Autodesk Fusion 360 part; units mm, degrees
(part 4 of 6)
sketch "Sketch9" plane through (0, -25, 0) normal (0, 1, 0) x (-1, 0, 0)
  line L0 (-171.5, 52) -> (-171.5, 84)
  line L1 (-171.5, 84) -> (-111.5, 84)
  line L2 (-111.5, 84) -> (-111.5, 52)
  line L3 (-111.5, 52) -> (-171.5, 52)
  line L4 (-109, 89) -> (-139, 89)
  line L5 (-139, 89) -> (-139, 142)
  line L6 (-139, 142) -> (-109, 142)
  line L7 (-109, 142) -> (-109, 89)
  line L8 (-174, 89) -> (-174, 142)
  line L9 (-174, 142) -> (-144, 142)
  line L10 (-144, 142) -> (-144, 89)
  line L11 (-144, 89) -> (-174, 89)
  line L12 (-96, 65.5) -> (-93, 65.5)
  line L13 (-93, 65.5) -> (-93, 128.5)
  line L14 (-93, 128.5) -> (-60, 128.5)
  line L15 (-60, 128.5) -> (-60, 65.5)
  line L16 (-60, 65.5) -> (-57, 65.5)
  line L17 (-57, 65.5) -> (-57, 130.6162)
  line L18 (-57, 130.6162) -> (-54, 130.6162)
  line L19 (-54, 130.6162) -> (-54, 62.5)
  line L20 (-54, 62.5) -> (-99, 62.5)
  line L21 (-99, 62.5) -> (-99, 130.6162)
  line L22 (-99, 130.6162) -> (-96, 130.6162)
  line L23 (-96, 130.6162) -> (-96, 65.5)
  arc A0 (-52, 27) -> (-44, 35) centre (-52, 35) ccw
  line L24 (-44, 35) -> (-44, 159)
  arc A1 (-44, 159) -> (-52, 167) centre (-52, 159) ccw
  line L25 (-52, 167) -> (-176, 167)
  arc A2 (-176, 167) -> (-184, 159) centre (-176, 159) ccw
  line L26 (-184, 159) -> (-184, 35)
  arc A3 (-184, 35) -> (-176, 27) centre (-176, 35) ccw
  line L27 (-176, 27) -> (-52, 27)
  line L28 (-134, 27) -> (-94, 27)
  line L29 (-94, 27) -> (-94, 33)
  line L30 (-94, 33) -> (-134, 33)
  line L31 (-134, 33) -> (-134, 27)
  dimension "d68" = 6
  dimension "d70" = 50
  dimension "d71" = 50
  dimension "d103" = 40
  constraint horizontal L28
  constraint vertical L29
  constraint horizontal L30
  constraint vertical L31
  constraint coincident L27 L28.start
  measures "d68" distance of L28.start L30.end
  measures "d70" distance of L26 L31
  measures "d71" distance of L24 L29
  measures "d103" distance of L29.end L30.end
extrude "Extrude10" cut sketch "Sketch9" against normal blind 4 contours L27 L28 L29 L30 L31
sketch "Sketch10" plane through (0, -25, 0) normal (0, 1, 0) x (-1, 0, 0)
  line L0 (-134, 27) -> (-134, 33)
  line L1 (-134, 33) -> (-94, 33)
  line L2 (-94, 33) -> (-94, 27)
  line L3 (-94, 27) -> (-52, 27)
  arc A0 (-52, 27) -> (-44, 35) centre (-52, 35) ccw
  line L4 (-44, 35) -> (-44, 159)
  arc A1 (-44, 159) -> (-52, 167) centre (-52, 159) ccw
  line L5 (-52, 167) -> (-176, 167)
  arc A2 (-176, 167) -> (-184, 159) centre (-176, 159) ccw
  line L6 (-184, 159) -> (-184, 35)
  arc A3 (-184, 35) -> (-176, 27) centre (-176, 35) ccw
  line L7 (-176, 27) -> (-134, 27)
  line L8 (-96, 65.5) -> (-93, 65.5)
  line L9 (-93, 65.5) -> (-93, 128.5)
  line L10 (-93, 128.5) -> (-60, 128.5)
  line L11 (-60, 128.5) -> (-60, 65.5)
  line L12 (-60, 65.5) -> (-57, 65.5)
  line L13 (-57, 65.5) -> (-57, 130.6162)
  line L14 (-57, 130.6162) -> (-54, 130.6162)
  line L15 (-54, 130.6162) -> (-54, 62.5)
  line L16 (-54, 62.5) -> (-99, 62.5)
  line L17 (-99, 62.5) -> (-99, 130.6162)
  line L18 (-99, 130.6162) -> (-96, 130.6162)
  line L19 (-96, 130.6162) -> (-96, 65.5)
  line L20 (-174, 89) -> (-174, 142)
  line L21 (-174, 142) -> (-144, 142)
  line L22 (-144, 142) -> (-144, 89)
  line L23 (-144, 89) -> (-174, 89)
  line L24 (-109, 89) -> (-139, 89)
  line L25 (-139, 89) -> (-139, 142)
  line L26 (-139, 142) -> (-109, 142)
  line L27 (-109, 142) -> (-109, 89)
  line L28 (-171.5, 52) -> (-171.5, 84)
  line L29 (-171.5, 84) -> (-111.5, 84)
  line L30 (-111.5, 84) -> (-111.5, 52)
  line L31 (-111.5, 52) -> (-171.5, 52)
  line L32 (-184, 37) -> (-44, 37)
  line L33 (-44, 37) -> (-44, 33)
  line L34 (-44, 33) -> (-184, 33)
  line L35 (-184, 33) -> (-184, 37)
  dimension "d74" = 4
  constraint horizontal L32
  constraint vertical L33
  constraint horizontal L34
  constraint vertical L35
  constraint collinear L1 L34
  constraint collinear L4 L33
  constraint collinear L6 L35
  measures "d74" distance of L32 L34
extrude "Extrude11" add sketch "Sketch10" along normal blind 19 contours L1 A0 L4 L6 A3 L32 L33 L34 L35 | A3 L34 L35 | A0 L33 L34
sketch "Sketch11" plane through (0, -23, 0) normal (0, 1, 0) x (-1, 0, 0)
  line L0 (-174, 89) -> (-144, 89)
  line L1 (-144, 89) -> (-144, 142)
  line L2 (-144, 142) -> (-174, 142)
  line L3 (-174, 142) -> (-174, 89)
  line L4 (-169, 142) -> (-149, 142)
  line L5 (-149, 142) -> (-149, 132)
  line L6 (-149, 132) -> (-169, 132)
  line L7 (-169, 132) -> (-169, 142)
  line L8 (-134, 132) -> (-114, 132)
  line L9 (-114, 132) -> (-114, 142)
  line L10 (-114, 142) -> (-134, 142)
  line L11 (-134, 142) -> (-134, 132)
  line L12 (-171.5, 74) -> (-161.5, 74)
  line L13 (-161.5, 74) -> (-161.5, 62)
  line L14 (-161.5, 62) -> (-171.5, 62)
  line L15 (-171.5, 62) -> (-171.5, 74)
  line L16 (-171.5, 84) -> (-171.5, 52)
  line L17 (-111.5, 84) -> (-171.5, 84)
  line L18 (-171.5, 52) -> (-111.5, 52)
  line L19 (-111.5, 52) -> (-111.5, 84)
  line L20 (-111.5, 84) -> (-171.5, 84)
  line L21 (-171.5, 84) -> (-171.5, 52)
  line L22 (-109, 142) -> (-139, 142)
  line L23 (-109, 89) -> (-109, 142)
  line L24 (-139, 142) -> (-139, 89)
  dimension "d93" = 10
  dimension "d94" = 10
  dimension "d95" = 10
  dimension "d96" = 5
  dimension "d97" = 5
  dimension "d98" = 10
  dimension "d100" = 10
  dimension "d101" = 5
  dimension "d102" = 5
  constraint horizontal L4
  constraint vertical L5
  constraint horizontal L6
  constraint vertical L7
  constraint horizontal L8
  constraint vertical L9
  constraint horizontal L10
  constraint vertical L11
  constraint horizontal L12
  constraint vertical L13
  constraint horizontal L14
  constraint vertical L15
  constraint collinear L15 L16
  constraint collinear L4 L10
  constraint collinear L2 L4
  measures "d93" distance of L12.start L12.end
  measures "d94" distance of L12 L17
  measures "d95" distance of L14 L18
  measures "d96" distance of L1 L5
  measures "d97" distance of L3 L7
  measures "d98" distance of L4.end L5.end
  measures "d100" distance of L8 L22
  measures "d101" distance of L9 L23
  measures "d102" distance of L11 L24
extrude "Extrude12" cut sketch "Sketch11" against normal blind 6 contours L2 L4 L5 L6 L7 | L8 L9 L10 L11 L22 | L12 L13 L14 L15 L16 L21
sketch "Sketch12" plane through (0, -21, 0) normal (0, 1, 0) x (-1, 0, 0)
  line L0 (-57, 65.5) -> (-96, 65.5)
  line L1 (-96, 65.5) -> (-96, 130.6162)
  line L2 (-96, 130.6162) -> (-99, 130.6162)
  line L3 (-99, 130.6162) -> (-99, 62.5)
  line L4 (-99, 62.5) -> (-54, 62.5)
  line L5 (-54, 62.5) -> (-54, 130.6162)
  line L6 (-54, 130.6162) -> (-57, 130.6162)
  line L7 (-57, 130.6162) -> (-57, 65.5)
  line L8 (-99, 62.5) -> (-54, 62.5)
  line L9 (-54, 62.5) -> (-54, 75.5)
  line L10 (-54, 75.5) -> (-99, 75.5)
  line L11 (-99, 75.5) -> (-99, 62.5)
  dimension "d79" = 10
  constraint horizontal L8
  constraint vertical L9
  constraint horizontal L10
  constraint vertical L11
  constraint coincident L5 L9.end
  constraint coincident L3.end L4.start
  measures "d79" distance of L0 L10
extrude "Extrude13" add sketch "Sketch12" against normal blind 1 contours L0 L1 L3 L4 L5 L7 L8 L9 L10 L11 | L0 L1 L7 L10
sketch "Sketch13" plane through (0, -21, 0) normal (0, 1, 0) x (-1, 0, 0)
  line L0 (-54, 62.5) -> (-54, 130.6162)
  line L1 (-54, 130.6162) -> (-57, 130.6162)
  line L2 (-57, 130.6162) -> (-57, 75.5)
  line L3 (-57, 75.5) -> (-96, 75.5)
  line L4 (-96, 75.5) -> (-96, 130.6162)
  line L5 (-96, 130.6162) -> (-99, 130.6162)
  line L6 (-99, 130.6162) -> (-99, 62.5)
  line L7 (-99, 62.5) -> (-54, 62.5)
  line L8 (-99, 72) -> (-54, 72)
  line L9 (-54, 72) -> (-54, 70)
  line L10 (-54, 70) -> (-99, 70)
  line L11 (-99, 70) -> (-99, 72)
  dimension "d82" = 2
  constraint horizontal L8
  constraint vertical L9
  constraint horizontal L10
  constraint vertical L11
  constraint coincident L0 L9.end
  constraint coincident L6 L8.start
  measures "d82" distance of L8.end L9.end
extrude "Extrude14" add sketch "Sketch13" along normal blind 6 contours L0 L6 L8 L9 L10 L11
equation "d1 = 184 mm + ( ( 12 / 2 ) * 1 mm )"
equation "d2 = 140 mm + ( ( 2 * 27 ) * 1 mm )"
equation "d24 = 7.25 mm + ( ( 5.5 / 2 ) * 1 mm )"
equation "d25 = 7.25 mm + ( ( 5.5 / 2 ) * 1 mm )"
equation "d55 = ( ( 39 - 33 ) / 2 ) * 1 mm"
equation "d56 = ( ( 39 - 33 ) / 2 ) * 1 mm"
named bodies: "Electronics Holder"

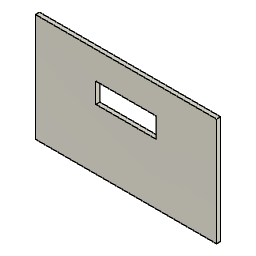
design "Unsorted Smarties Back Panel"
Autodesk Fusion 360 part; units mm, degrees
sketch "Unsorted Smarties Back" plane through (0, 0, 0) normal (0, 1, 0) x (1, 0, 0)
  line L0 (0, 0) -> (270, 0)
  line L1 (270, 0) -> (270, -161)
  line L2 (270, -161) -> (0, -161)
  line L3 (0, -161) -> (0, 0)
  dimension "d1" = 270
  dimension "d2" = 161
  constraint horizontal L0
  constraint vertical L1
  constraint horizontal L2
  constraint vertical L3
  constraint coincident L0.start L3.end
  measures "d1" distance of L0.start L0.end
  measures "d2" distance of L0.end L1.end
extrude "Extrude1" add sketch "Unsorted Smarties Back" along normal blind 6
sketch "Smartie Feed" plane through (0, 0, 0) normal (0, -1, 0) x (1, 0, 0)
  line L0 (270, 161) -> (0, 161)
  line L1 (0, 161) -> (0, 0)
  line L2 (0, 0) -> (270, 0)
  line L3 (270, 0) -> (270, 161)
  line L4 (90, 120) -> (180, 120)
  line L5 (180, 120) -> (180, 90)
  line L6 (180, 90) -> (90, 90)
  line L7 (90, 90) -> (90, 120)
  dimension "d6" = 90
  dimension "d7" = 90
  dimension "d8" = 41
  dimension "d9" = 30
  dimension "d12" = 90
  constraint horizontal L4
  constraint vertical L5
  constraint horizontal L6
  constraint vertical L7
  measures "d6" distance of L1 L7
  measures "d7" distance of L3 L5
  measures "d8" distance of L0 L4
  measures "d9" distance of L4.end L5.end
  measures "d12" distance of L5 L7
extrude "Extrude2" cut sketch "Smartie Feed" against normal blind 6 contours L4 L5 L6 L7
equation "mdfThickness = 6 mm"
equation "d4 = mdfThickness"
named bodies: "Unsorted Smarties Back Panel"

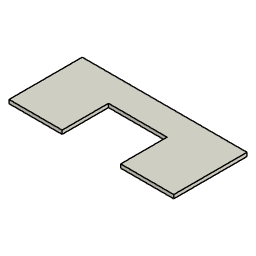
design "Colour Detection Mechanism Top Panel"
part number: 2025-05-13-09-48-31-121
Autodesk Fusion 360 part; units mm, degrees
sketch "Sorting Mechanism Top Panel" plane through (0, 0, 0) normal (0, 0, 1) x (1, 0, 0)
  line L0 (0, 0) -> (270, 0)
  line L1 (270, 0) -> (270, 120)
  line L2 (270, 120) -> (0, 120)
  line L3 (0, 120) -> (0, 0)
  dimension "d1" = 270
  dimension "d2" = 120
  constraint horizontal L0
  constraint vertical L1
  constraint horizontal L2
  constraint vertical L3
  constraint coincident L0.start L3.end
  measures "d1" distance of L0.start L0.end
  measures "d2" distance of L0.end L1.end
extrude "Extrude1" add sketch "Sorting Mechanism Top Panel" along normal blind 6
sketch "Smartie Hopper Hole" plane through (0, 0, 6) normal (0, 0, 1) x (-1, 0, 0)
  line L0 (0, -120) -> (0, 0)
  line L1 (0, 0) -> (-270, 0)
  line L2 (-270, 0) -> (-270, -120)
  line L3 (-270, -120) -> (0, -120)
  line L4 (-87, -76) -> (-183, -76)
  line L5 (-183, -76) -> (-183, 0)
  line L6 (-183, 0) -> (-87, 0)
  line L7 (-87, 0) -> (-87, -76)
  dimension "d7" = 96
  dimension "d9" = 76
  dimension "d10" = 87
  dimension "d11" = 87
  constraint horizontal L4
  constraint vertical L5
  constraint horizontal L6
  constraint vertical L7
  constraint collinear L1 L6
  measures "d7" distance of L4.start L4.end
  measures "d9" distance of L4.end L5.end
  measures "d10" distance of L0 L7
  measures "d11" distance of L2 L5
extrude "Extrude2" cut sketch "Smartie Hopper Hole" against normal blind 6 contours L1 L4 L5 L6 L7
equation "d3 = MDF_thickness"
equation "acrylic_thickness = 3 mm"
equation "MDF_thickness = 6 mm"
equation "d7 = smarties_hopper_width + 2 * acrylic_thickness"
equation "smarties_hopper_width = 90 mm"
equation "d9 = smarties_hopper_depth + 2 * acrylic_thickness"
equation "d10 = ( 270 mm - ( smarties_hopper_width + 2 * acrylic_thickness ) ) / 2"
equation "smarties_hopper_depth = 70 mm"
named bodies: "Sorting Mechanism Top Panel"

design "5 Volt Label"
Autodesk Fusion 360 part; units mm, degrees
sketch "Sticker" plane through (0, 0, 0) normal (0, 1, 0) x (1, 0, 0)
  line L0 (0, 0) -> (15, 0)
  line L1 (15, 0) -> (15, -12)
  line L2 (15, -12) -> (0, -12)
  line L3 (0, -12) -> (0, 0)
  dimension "d1" = 12
  dimension "d2" = 15
  constraint horizontal L0
  constraint vertical L1
  constraint horizontal L2
  constraint vertical L3
  constraint coincident L0.start L3.end
  measures "d1" distance of L0.end L1.end
  measures "d2" distance of L0.start L0.end
extrude "Extrude1" add sketch "Sticker" along normal blind 0.01 makes body 1
sketch "Text" plane through (0, 0, 0) normal (0, -1, 0) x (1, 0, 0)
  line L0 (15, 12) -> (0, 12)
  line L1 (0, 12) -> (0, 0)
  line L2 (0, 0) -> (15, 0)
  line L3 (15, 0) -> (15, 12)
  line L4 (0, 0) -> (15, 0) construction
  line L5 (15, 0) -> (15, 12) construction
  line L6 (15, 12) -> (0, 12) construction
  line L7 (0, 12) -> (0, 0) construction
  dimension "d5" = 5
  dimension "d8" = 0
  text T0 "5 V" font "Arial" height 5 align centre middle in box 15 x 12 at (0, 0) x (1, 0) y (0, 1) spacing 1 kerned
  constraint coincident L2.end
  constraint coincident L0.end
extrude "Extrude2" add sketch "Text" along normal blind 0.01 separate body text T0 makes body 2 at (4.016, 0, 8.2362) makes body 3 at (8.9069, 0, 7.2892)
equation "d8 = '5 V'"

design "Top Access Panel"
Autodesk Fusion 360 part; units mm, degrees
sketch "Top Access Panel" plane through (0, 0, 0) normal (0, 1, 0) x (1, 0, 0)
  line L0 (0, 0) -> (119, 0)
  line L1 (119, 0) -> (119, -89)
  line L2 (119, -89) -> (0, -89)
  line L3 (0, -89) -> (0, 0)
  dimension "d1" = 119
  dimension "d2" = 89
  constraint horizontal L0
  constraint vertical L1
  constraint horizontal L2
  constraint vertical L3
  constraint coincident L0.start L3.end
  measures "d1" distance of L0.start L0.end
  measures "d2" distance of L0.end L1.end
extrude "Extrude1" add sketch "Top Access Panel" along normal blind 6
fillet "Fillet1" radius 8 4 edges at (0, 3, 89) (119, 3, 89) (119, 3, 0) (0, 3, 0)
sketch "Handle" plane through (0, 6, 0) normal (0, 1, 0) x (-1, 0, 0)
  arc A0 (-8, 0) -> (0, 8) centre (-8, 8) ccw
  line L0 (0, 8) -> (0, 81)
  arc A1 (0, 81) -> (-8, 89) centre (-8, 81) ccw
  line L1 (-8, 89) -> (-111, 89)
  arc A2 (-111, 89) -> (-119, 81) centre (-111, 81) ccw
  line L2 (-119, 81) -> (-119, 8)
  arc A3 (-119, 8) -> (-111, 0) centre (-111, 8) ccw
  line L3 (-111, 0) -> (-8, 0)
  line L4 (-99, 0) -> (-20, 0)
  line L5 (-20, 0) -> (-20, 15)
  line L6 (-20, 15) -> (-99, 15)
  line L7 (-99, 15) -> (-99, 0)
  dimension "d16" = 15
  dimension "d17" = 20
  dimension "d18" = 20
  constraint horizontal L4
  constraint vertical L5
  constraint horizontal L6
  constraint vertical L7
  measures "d16" distance of L4 L6
  measures "d17" distance of L2 L7
  measures "d18" distance of L0 L5
extrude "Extrude3" cut sketch "Handle" against normal blind 6 contours L3 L4 L5 L6 L7
fillet "Fillet2" radius 15 2 edges at (99, 3, 15) (20, 3, 15)
sketch "Sketch4" plane through (0, 0, 0) normal (0, -1, 0) x (1, 0, 0)
  line L0 (35, 15) -> (84, 15)
  arc A0 (99, 0) -> (84, 15) centre (84, 0) ccw
  line L1 (99, 0) -> (111, 0)
  arc A1 (111, 0) -> (119, 8) centre (111, 8) ccw
  line L2 (119, 8) -> (119, 81)
  arc A2 (119, 81) -> (111, 89) centre (111, 81) ccw
  line L3 (111, 89) -> (8, 89)
  arc A3 (8, 89) -> (0, 81) centre (8, 81) ccw
  line L4 (0, 81) -> (0, 8)
  arc A4 (0, 8) -> (8, 0) centre (8, 8) ccw
  line L5 (8, 0) -> (20, 0)
  arc A5 (35, 15) -> (20, 0) centre (35, 0) ccw
  circle A6 centre (9.5, 79.237) radius 2.75
  circle A7 centre (109.5, 79.237) radius 2.75
  circle A8 centre (9.5, 9.237) radius 2.75
  circle A9 centre (109.5, 9.237) radius 2.75
  dimension "d23" = 5.5
  dimension "d24" = 5.5
  dimension "d25" = 5.5
  dimension "d26" = 5.5
  dimension "d27" = 9.5
  dimension "d28" = 9.5
  dimension "d29" = 9.5
  dimension "d30" = 9.5
  dimension "d31" = 9.763
  dimension "d32" = 9.763
  dimension "d33" = 9.237
  dimension "d34" = 9.237
  measures "d23" diameter of A6
  measures "d24" diameter of A7
  measures "d25" diameter of A8
  measures "d26" diameter of A9
  measures "d27" distance of L2 A9.centre
  measures "d28" distance of L4 A8.centre
  measures "d29" distance of L4 A6.centre
  measures "d30" distance of L2 A7.centre
  measures "d31" distance of L3 A6.centre
  measures "d32" distance of L3 A7.centre
  measures "d33" distance of L5 A8.centre
  measures "d34" distance of L1 A9.centre
extrude "Extrude4" cut sketch "Sketch4" against normal blind 1.5 contours A6 | A7 | A8 | A9
equation "mdfThickness = 6 mm"
equation "d4 = mdfThickness"
equation "filletRadius = 8 mm"
equation "d15 = filletRadius"
equation "d27 = 7.5 mm + ( ( 5.5 / 2 ) * 1 mm ) - 0.25 mm - 0.5 mm"
equation "d28 = 7.5 mm + ( ( 5.5 / 2 ) * 1 mm ) - 0.25 mm - 0.5 mm"
equation "d29 = 7.5 mm + ( ( 5.5 / 2 ) * 1 mm ) - 0.25 mm - 0.5 mm"
equation "d30 = 7.5 mm + ( ( 5.5 / 2 ) * 1 mm ) - 0.25 mm - 0.5 mm"
equation "d31 = 7.763 mm + ( ( 5.5 / 2 ) * 1 mm ) - 0.25 mm - 0.5 mm"
equation "d32 = 7.763 mm + ( ( 5.5 / 2 ) * 1 mm ) - 0.25 mm - 0.5 mm"
equation "d33 = 7.237 mm + ( ( 5.5 / 2 ) * 1 mm ) - 0.25 mm - 0.5 mm"
equation "d34 = 7.237 mm + ( ( 5.5 / 2 ) * 1 mm ) - 0.25 mm - 0.5 mm"

design "Name Sign Conduit"
Autodesk Fusion 360 part; units mm, degrees
sketch "16 mm x 16 mm conduit piping shape" plane through (0, 0, 0) normal (1, 0, 0) x (0, 1, 0)
  line L0 (0, 0) -> (16, 0)
  line L1 (16, 0) -> (16, 10)
  line L2 (16, 10) -> (14, 13.9)
  line L3 (14, 13.9) -> (13.1102, 13.4437)
  line L4 (13.1102, 13.4437) -> (15, 9.7585)
  line L5 (15, 9.7585) -> (15, 1)
  line L6 (15, 1) -> (1, 1)
  line L7 (1, 1) -> (1, 9.7585)
  line L8 (1, 9.7585) -> (2.8898, 13.4437)
  line L9 (2.8898, 13.4437) -> (2, 13.9)
  line L10 (2, 13.9) -> (0, 10)
  line L11 (0, 10) -> (0, 0)
  line L12 (0, 16) -> (16, 16)
  line L13 (0, 16) -> (0, 12)
  line L14 (0, 12) -> (1, 12)
  line L15 (1, 12) -> (1, 15)
  line L16 (1, 15) -> (15, 15)
  line L17 (15, 15) -> (15, 12)
  line L18 (15, 12) -> (16, 12)
  line L19 (16, 12) -> (16, 16)
  dimension "d1" = 1
  dimension "d2" = 16
  dimension "d3" = 1
  dimension "d4" = 1
  dimension "d7" = 10
  dimension "d8" = 10
  dimension "d9" = 16
  dimension "d10" = 1
  dimension "d11" = 1
  dimension "d12" = 1
  dimension "d13" = 4
  dimension "d14" = 4
  dimension "d15" = 16
  dimension "d16" = 2
  dimension "d17" = 2
  dimension "d18" = 1
  dimension "d19" = 1
  constraint coincident L0.start L11.end
  constraint horizontal L0
  constraint perpendicular L0 L1
  constraint perpendicular L2 L3
  constraint parallel L1 L5
  constraint perpendicular L5 L6
  constraint perpendicular L6 L7
  constraint perpendicular L0 L11
  constraint horizontal L12
  constraint perpendicular L12 L13
  constraint perpendicular L13 L14
  constraint perpendicular L14 L15
  constraint perpendicular L15 L16
  constraint perpendicular L16 L17
  constraint perpendicular L17 L18
  constraint perpendicular L12 L19
  constraint parallel L8 L10
  constraint parallel L2 L4
  constraint perpendicular L9 L10
  measures "d1" distance of L0 L6
  measures "d2" distance of L1 L11
  measures "d3" distance of L7 L11
  measures "d4" distance of L1 L5
  measures "d7" distance of L0.end L1.end
  measures "d8" distance of L10.end L0.start
  measures "d9" distance of L0 L12
  measures "d10" distance of L12 L16
  measures "d11" distance of L17 L19
  measures "d12" distance of L13 L15
  measures "d13" distance of L12.end L18.end
  measures "d14" distance of L12.start L13.end
  measures "d15" distance of L12.start L12.end
  measures "d16" distance of L1.end L2.end
  measures "d17" distance of L9.end L10.end
  measures "d18" distance of L2.end L3.end
  measures "d19" distance of L8.end L9.end
extrude "Extrude1" add sketch "16 mm x 16 mm conduit piping shape" along normal blind 161 makes body 1 at (107.3333, 5.3333, 16) makes body 2 at (53.6667, 5.3333, 0)
fillet "Fillet1" radius 0.3 18 edges at (80.5, 0, 16) (80.5, 16, 16) (80.5, 16, 12) (80.5, 0, 12) (80.5, 1, 12) (80.5, 15, 12) (80.5, 1, 15) (80.5, 15, 15) (80.5, 0, 10) (80.5, 16, 10) (80.5, 14, 13.9) (80.5, 13.1102, 13.4437) (80.5, 2, 13.9) (80.5, 2.8898, 13.4437) (80.5, 15, 1) (80.5, 1, 1) (80.5, 1, 9.7585) (80.5, 15, 9.7585) on bodies 1 2
equation "d1 = conduitThickness"
equation "d2 = conduitWidth"
equation "d3 = conduitThickness"
equation "d4 = conduitThickness"
equation "conduitThickness = 1 mm"
equation "conduitWidth = 16 mm"
equation "d9 = conduitWidth"
equation "d10 = conduitThickness"
equation "d11 = conduitThickness"
equation "d12 = conduitThickness"

design "Bottom Panel Opener"
Autodesk Fusion 360 part; units mm, degrees
sketch "Sketch1" plane through (0, 0, 0) normal (0, 0, 1) x (1, 0, 0)
  line L0 (-47.9346, 62.0575) -> (-70.9346, 62.0575)
  line L1 (-70.9346, 62.0575) -> (-70.9346, 122.0575)
  line L2 (-70.9346, 122.0575) -> (-47.9346, 122.0575)
  line L3 (-47.9346, 122.0575) -> (-47.9346, 62.0575)
  line L4 (-70.9346, 110) -> (-94.9346, 110)
  line L5 (-94.9346, 110) -> (-94.9346, 75)
  line L6 (-94.9346, 75) -> (-70.9346, 75)
  line L7 (-70.9346, 75) -> (-70.9346, 110)
  dimension "d1" = 35
  dimension "d3" = 60
  dimension "d4" = 24
  dimension "d10" = 23
  constraint horizontal L0
  constraint vertical L1
  constraint horizontal L2
  constraint vertical L3
  constraint horizontal L4
  constraint vertical L5
  constraint horizontal L6
  constraint vertical L7
  constraint coincident L1 L4.start
  measures "d1" distance of L4.end L5.end
  measures "d3" distance of L0.start L2.end
  measures "d4" distance of L4.start L4.end
  measures "d10" distance of L1 L3
extrude "Extrude1" add sketch "Sketch1" along normal blind 4
fillet "Fillet1" radius 4 2 edges at (-47.9346, 62.0575, 2) (-47.9346, 122.0575, 2)
fillet "Fillet1" radius 4 2 edges at (-94.9346, 75, 2) (-94.9346, 110, 2)

design "Front Panel"
Autodesk Fusion 360 part; units mm, degrees
sketch "Front Panel" plane through (0, 0, 0) normal (0, 1, 0) x (1, 0, 0)
  line L0 (0, 0) -> (270, 0)
  line L1 (270, 0) -> (270, -30)
  line L2 (258, -16) -> (12, -16)
  line L3 (0, -59) -> (0, 0)
  line L4 (12, -16) -> (12, -59)
  line L5 (12, -59) -> (0, -59)
  line L6 (258, -16) -> (258, -59)
  line L7 (258, -59) -> (270, -59)
  line L8 (270, -59) -> (270, -30)
  dimension "d1" = 270
  dimension "d3" = 43
  dimension "d4" = 12
  dimension "d5" = 12
  dimension "d10" = 16
  dimension "d11" = 43
  constraint horizontal L0
  constraint vertical L1
  constraint horizontal L2
  constraint vertical L3
  constraint coincident L0.start L3.end
  constraint vertical L4
  constraint horizontal L5
  constraint vertical L6
  constraint horizontal L7
  constraint vertical L8
  measures "d1" distance of L0.start L0.end
  measures "d3" distance of L2.end L4.end
  measures "d4" distance of L6.end L7.end
  measures "d5" distance of L4.end L3.start
  measures "d10" distance of L0 L2
  measures "d11" distance of L2 L7
extrude "Extrude1" add sketch "Front Panel" along normal blind 6
equation "mdfThickness = 6 mm"
equation "d7 = mdfThickness"
equation "d10 = 10 mm + mdfThickness"

design "Name Sign Bottom Connector"
Autodesk Fusion 360 part; units mm, degrees
sketch "Sketch1" plane through (0, 0, 0) normal (1, 0, 0) x (0, 1, 0)
  line L0 (25, 0) -> (0, 0)
  line L1 (0, 0) -> (-23.1302, 9.4864)
  line L2 (-23.1302, 9.4864) -> (-22.3713, 11.3368)
  line L3 (-22.3713, 11.3368) -> (0.3942, 2)
  line L4 (0.3942, 2) -> (25, 2)
  line L5 (25, 2) -> (25, 0)
  dimension "d1" = 157.7
  dimension "d2" = 2
  dimension "d3" = 2
  dimension "d4" = 25
  dimension "d5" = 25
  constraint coincident L0.end L1.start
  constraint horizontal L0
  constraint perpendicular L1 L2
  constraint perpendicular L2 L3
  constraint horizontal L4
  constraint perpendicular L0 L5
  measures "d1" angle of L3 L4
  measures "d2" distance of L0.start L4.end
  measures "d3" distance of L1.end L2.end
  measures "d4" distance of L0.end L1.end
  measures "d5" distance of L0.start L0.end
extrude "Extrude1" add sketch "Sketch1" against normal blind 15
sketch "Sketch2" plane through (0, 0, 2) normal (0, 0, 1) x (-1, 0, 0)
  line L0 (0, -0.3942) -> (0, -25)
  line L1 (0, -25) -> (15, -25)
  line L2 (15, -25) -> (15, -0.3942)
  line L3 (15, -0.3942) -> (0, -0.3942)
  circle A0 centre (5, -7.3942) radius 3
  circle A1 centre (10, -18) radius 3
  dimension "d8" = 6
  dimension "d9" = 6
  dimension "d10" = 5
  dimension "d11" = 5
  dimension "d12" = 7
  dimension "d14" = 7
  measures "d8" diameter of A0
  measures "d9" diameter of A1
  measures "d10" distance of L2 A1.centre
  measures "d11" distance of L0 A0.centre
  measures "d12" distance of L1 A1.centre
  measures "d14" distance of L3 A0.centre
sketch "Sketch3" plane through (0, 0.7589, 1.8504) normal (0, 0.379456, 0.92521) x (-1, 0, 0)
  line L0 (0, 25) -> (0, 0.3942)
  line L1 (0, 0.3942) -> (15, 0.3942)
  line L2 (15, 0.3942) -> (15, 25)
  line L3 (15, 25) -> (0, 25)
  circle A0 centre (10, 7.3942) radius 3
  circle A1 centre (5, 18) radius 3
  dimension "d15" = 6
  dimension "d16" = 6
  dimension "d17" = 5
  dimension "d18" = 5
  dimension "d19" = 7
  dimension "d20" = 7
  measures "d15" diameter of A0
  measures "d16" diameter of A1
  measures "d17" distance of L0 A1.centre
  measures "d18" distance of L2 A0.centre
  measures "d19" distance of L3 A1.centre
  measures "d20" distance of L1 A0.centre
extrude "Extrude2" cut sketch "Sketch3" against normal blind 2 contours A0 | A1
extrude "Extrude3" cut sketch "Sketch2" against normal blind 2 contours A0 | A1
fillet "Fillet1" radius 0.3 8 edges at (-2.203, -16.8986, 9.0923) (-7.203, -7.086, 5.0678) (-2.203, 6.3094, 2) (-7.203, 16.9152, 2) (-2.203, -15.6501, 6.4186) (-7.203, -5.8375, 2.3941) (-2.203, 8.479, 0) (-7.203, 19.0848, 0)

design "Smartie Arm"
Autodesk Fusion 360 part; units mm, degrees
sketch "Smartie Arm" plane through (0, 0, 0) normal (0, 0, 1) x (1, 0, 0)
  line L0 (0, 0) -> (95, 0)
  line L1 (95, 0) -> (95, 95)
  line L2 (95, 95) -> (0, 95)
  line L3 (0, 95) -> (0, 0)
  dimension "d6" = 95
  dimension "d15" = 95
  constraint horizontal L0
  constraint vertical L1
  constraint horizontal L2
  constraint vertical L3
  constraint coincident L0.start L3.end
  measures "d6" distance of L1.end L2.end
  measures "d15" distance of L0.end L1.end
extrude "Extrude1" add sketch "Smartie Arm" along normal blind 8
sketch "Smartie Hole" plane through (0, 0, 8) normal (0, 0, 1) x (-1, 0, 0)
  line L0 (0, -95) -> (0, 0)
  line L1 (0, 0) -> (-95, 0)
  line L2 (-95, 0) -> (-95, -95)
  line L3 (-95, -95) -> (0, -95)
  circle A0 centre (-15, -81) radius 9
  dimension "d5" = 18
  dimension "d8" = 15
  dimension "d9" = 80
  dimension "d14" = 14
  measures "d5" diameter of A0
  measures "d8" distance of L0 A0.centre
  measures "d9" distance of L2 A0.centre
  measures "d14" distance of L3 A0.centre
extrude "Extrude2" cut sketch "Smartie Hole" against normal blind 8 contours A0
fillet "Fillet1" radius 15 2 edges at (95, 95, 4) (0, 95, 4)
fillet "Fillet2" radius 15 2 edges at (0, 0, 4) (95, 0, 4)
sketch "Smartie Arm Arc" plane through (0, 0, 8) normal (0, 0, 1) x (-1, 0, 0)
  arc A0 (-80, 0) -> (-95, -15) centre (-80, -15) ccw
  line L0 (-95, -15) -> (-95, -80)
  arc A1 (-95, -80) -> (-80, -95) centre (-80, -80) ccw
  line L1 (-80, -95) -> (-15, -95)
  arc A2 (-15, -95) -> (0, -80) centre (-15, -80) ccw
  line L2 (0, -80) -> (0, -15)
  arc A3 (0, -15) -> (-15, 0) centre (-15, -15) ccw
  line L3 (-15, 0) -> (-80, 0)
  circle A4 centre (-15, -81) radius 9
  circle A5 centre (-15, -15) radius 80
  dimension "d16" = 15
  dimension "d17" = 15
  dimension "d18" = 160
  measures "d16" distance of L2.end A3.centre
  measures "d17" distance of L3 A3.centre
  measures "d18" diameter of A5
extrude "Extrude3" cut sketch "Smartie Arm Arc" against normal blind 8 contours L0 A1 L1 A5
equation "d14 = 16 mm - 2 mm"

design "Back Panel Support Bottom"
Autodesk Fusion 360 part; units mm, degrees
sketch "Back Panel Support Left " plane through (0, 0, 0) normal (1, 0, 0) x (0, 1, 0)
  line L0 (0, 0) -> (21, 0)
  line L1 (21, 0) -> (21, 21)
  line L2 (21, 21) -> (0, 21)
  line L3 (0, 21) -> (0, 0)
  dimension "d1" = 21
  dimension "d2" = 21
  constraint horizontal L0
  constraint vertical L1
  constraint horizontal L2
  constraint vertical L3
  constraint coincident L0.start L3.end
  measures "d1" distance of L0.end L1.end
  measures "d2" distance of L0.start L0.end
extrude "Extrude1" add sketch "Back Panel Support Left " along normal blind 228

design "Bottom Label"
Autodesk Fusion 360 part; units mm, degrees
sketch "Sticker" plane through (0, 0, 0) normal (0, 1, 0) x (1, 0, 0)
  line L0 (0, 0) -> (45, 0)
  line L1 (45, 0) -> (45, -12)
  line L2 (45, -12) -> (0, -12)
  line L3 (0, -12) -> (0, 0)
  dimension "d1" = 12
  dimension "d2" = 45
  constraint horizontal L0
  constraint vertical L1
  constraint horizontal L2
  constraint vertical L3
  constraint coincident L0.start L3.end
  measures "d1" distance of L0.end L1.end
  measures "d2" distance of L0.start L0.end
extrude "Extrude1" add sketch "Sticker" along normal blind 0.01 makes body 1
sketch "Text" plane through (0, 0, 0) normal (0, -1, 0) x (1, 0, 0)
  line L0 (45, 12) -> (0, 12)
  line L1 (0, 12) -> (0, 0)
  line L2 (0, 0) -> (45, 0)
  line L3 (45, 0) -> (45, 12)
  line L4 (0, 0) -> (45, 0) construction
  line L5 (45, 0) -> (45, 12) construction
  line L6 (45, 12) -> (0, 12) construction
  line L7 (0, 12) -> (0, 0) construction
  dimension "d5" = 5
  text T0 "Bottom" font "Arial" height 5 align centre middle in box 45 x 12 at (0, 0) x (1, 0) y (0, 1) spacing 1 kerned
  constraint coincident L2.end
  constraint coincident L0.end
extrude "Extrude2" add sketch "Text" along normal blind 0.01 separate body text T0 makes body 2 at (16.525, 0, 5.5613) makes body 3 at (28.3799, 0, 5.3338) makes body 4 at (24.291, 0, 5.5613) makes body 5 at (22.8695, 0, 5.244) makes body 6 at (20.9288, 0, 5.244) makes body 7 at (12.1373, 0, 5.9363)

design "6 Volt Label"
Autodesk Fusion 360 part; units mm, degrees
sketch "Sticker" plane through (0, 0, 0) normal (0, 1, 0) x (1, 0, 0)
  line L0 (0, 0) -> (15, 0)
  line L1 (15, 0) -> (15, -12)
  line L2 (15, -12) -> (0, -12)
  line L3 (0, -12) -> (0, 0)
  dimension "d1" = 12
  dimension "d2" = 15
  constraint horizontal L0
  constraint vertical L1
  constraint horizontal L2
  constraint vertical L3
  constraint coincident L0.start L3.end
  measures "d1" distance of L0.end L1.end
  measures "d2" distance of L0.start L0.end
extrude "Extrude1" add sketch "Sticker" along normal blind 0.01 makes body 1
sketch "Text" plane through (0, 0, 0) normal (0, -1, 0) x (1, 0, 0)
  line L0 (15, 12) -> (0, 12)
  line L1 (0, 12) -> (0, 0)
  line L2 (0, 0) -> (15, 0)
  line L3 (15, 0) -> (15, 12)
  line L4 (0, 0) -> (15, 0) construction
  line L5 (15, 0) -> (15, 12) construction
  line L6 (15, 12) -> (0, 12) construction
  line L7 (0, 12) -> (0, 0) construction
  dimension "d5" = 5
  dimension "d8" = 0
  text T0 "6 V" font "Arial" height 5 align centre middle in box 15 x 12 at (0, 0) x (1, 0) y (0, 1) spacing 1 kerned
  constraint coincident L2.end
  constraint coincident L0.end
extrude "Extrude2" add sketch "Text" along normal blind 0.01 separate body text T0 makes body 2 at (2.6313, 0, 6.1669) makes body 3 at (8.9205, 0, 7.2892)
equation "d8 = 6 V"

design "Female Header Pins"
Autodesk Fusion 360 part; units mm, degrees
sketch "Plastic casing" plane through (0, 0, 0) normal (0, 1, 0) x (1, 0, 0)
  line L0 (0, 0) -> (2.54, 0)
  line L1 (2.54, 0) -> (2.54, -8)
  line L2 (2.54, -8) -> (0, -8)
  line L3 (0, -8) -> (0, 0)
  dimension "d1" = 8
  dimension "d2" = 2.54
  constraint horizontal L0
  constraint vertical L1
  constraint horizontal L2
  constraint vertical L3
  constraint coincident L0.start L3.end
  measures "d1" distance of L0.end L1.end
  measures "d2" distance of L0.start L0.end
extrude "Extrude1" add sketch "Plastic casing" along normal blind 2.5 makes body 1
sketch "Hole" plane through (0, 0, 8) normal (0, 0, 1) x (-1, 0, 0)
  line L0 (0, 0) -> (-2.54, 0)
  line L1 (-2.54, 0) -> (-2.54, -2.5)
  line L2 (-2.54, -2.5) -> (0, -2.5)
  line L3 (0, -2.5) -> (0, 0)
  line L4 (-0.5, -2) -> (-2.04, -2)
  line L5 (-2.04, -2) -> (-2.04, -0.5)
  line L6 (-2.04, -0.5) -> (-0.5, -0.5)
  line L7 (-0.5, -0.5) -> (-0.5, -2)
  dimension "d6" = 0.5
  dimension "d7" = 0.5
  dimension "d8" = 0.5
  dimension "d9" = 0.5
  constraint horizontal L4
  constraint vertical L5
  constraint horizontal L6
  constraint vertical L7
  measures "d6" distance of L2 L4
  measures "d7" distance of L0 L6
  measures "d8" distance of L3 L7
  measures "d9" distance of L1 L5
extrude "Extrude2" cut sketch "Hole" against normal blind 7 contours L4 L5 L6 L7 bodies 1
sketch "Pin" plane through (0, 0, 0) normal (0, 0, 1) x (1, 0, 0)
  line L0 (2.54, 0) -> (0, 0)
  line L1 (0, 0) -> (0, 2.5)
  line L2 (0, 2.5) -> (2.54, 2.5)
  line L3 (2.54, 2.5) -> (2.54, 0)
  line L4 (0.945, 1.09) -> (1.595, 1.09)
  line L5 (1.595, 1.09) -> (1.595, 1.41)
  line L6 (1.595, 1.41) -> (0.945, 1.41)
  line L7 (0.945, 1.41) -> (0.945, 1.09)
  dimension "d12" = 0.65
  dimension "d13" = 0.32
  dimension "d14" = 0.945
  dimension "d15" = 0.945
  dimension "d16" = 1.09
  dimension "d17" = 1.09
  constraint horizontal L4
  constraint vertical L5
  constraint horizontal L6
  constraint vertical L7
  measures "d12" distance of L5.end L6.end
  measures "d13" distance of L4.end L5.end
  measures "d14" distance of L1 L7
  measures "d15" distance of L3 L5
  measures "d16" distance of L2 L6
  measures "d17" distance of L0 L4
extrude "Extrude3" add sketch "Pin" against normal blind 12 separate body contours L4 L5 L6 L7 makes body 2
chamfer "Chamfer1" distance 0.2 distance2 2 2 edges at (1.595, 1.25, -12) (0.945, 1.25, -12) measured on face at (1.1617, 1.3033, -12) measured on face at (1.1617, 1.3033, -12) on bodies 2
pattern_linear "R-Pattern1" count 15 spacing 2.54 along (1, 0, 0) of bodies 1 2 makes body 3 at (3.3867, 0, 2.6667) makes body 4 at (5.9267, 0, 2.6667) makes body 5 at (8.4667, 0, 2.6667) makes body 6 at (11.0067, 0, 2.6667) makes body 7 at (13.5467, 0, 2.6667) makes body 8 at (16.0867, 0, 2.6667) makes body 9 at (18.6267, 0, 2.6667) makes body 10 at (21.1667, 0, 2.6667) makes body 11 at (23.7067, 0, 2.6667) makes body 12 at (26.2467, 0, 2.6667) makes body 13 at (28.7867, 0, 2.6667) makes body 14 at (31.3267, 0, 2.6667) makes body 15 at (33.8667, 0, 2.6667) makes body 16 at (36.4067, 0, 2.6667) makes body 17 at (3.9183, 1.41, -3.3333) makes body 18 at (6.4583, 1.41, -3.3333) makes body 19 at (8.9983, 1.41, -3.3333) makes body 20 at (11.5383, 1.41, -3.3333) makes body 21 at (14.0783, 1.41, -3.3333) makes body 22 at (16.6183, 1.41, -3.3333) makes body 23 at (19.1583, 1.41, -3.3333) makes body 24 at (21.6983, 1.41, -3.3333) makes body 25 at (24.2383, 1.41, -3.3333) makes body 26 at (26.7783, 1.41, -3.3333) makes body 27 at (29.3183, 1.41, -3.3333) makes body 28 at (31.6417, 1.09, -3.3333) makes body 29 at (34.3983, 1.41, -3.3333) makes body 30 at (36.9383, 1.41, -3.3333)
equation "d14 = ( ( 2.54 - 0.65 ) / 2 ) * 1 mm"
equation "d16 = ( ( 2.5 - 0.32 ) / 2 ) * 1 mm"

design "12 Volt Label"
Autodesk Fusion 360 part; units mm, degrees
sketch "Sticker" plane through (0, 0, 0) normal (0, 1, 0) x (1, 0, 0)
  line L0 (0, 0) -> (15, 0)
  line L1 (15, 0) -> (15, -12)
  line L2 (15, -12) -> (0, -12)
  line L3 (0, -12) -> (0, 0)
  dimension "d1" = 12
  dimension "d2" = 15
  constraint horizontal L0
  constraint vertical L1
  constraint horizontal L2
  constraint vertical L3
  constraint coincident L0.start L3.end
  measures "d1" distance of L0.end L1.end
  measures "d2" distance of L0.start L0.end
extrude "Extrude1" add sketch "Sticker" along normal blind 0.01 makes body 1
sketch "Text" plane through (0, 0, 0) normal (0, -1, 0) x (1, 0, 0)
  line L0 (15, 12) -> (0, 12)
  line L1 (0, 12) -> (0, 0)
  line L2 (0, 0) -> (15, 0)
  line L3 (15, 0) -> (15, 12)
  line L4 (0, 0) -> (15, 0) construction
  line L5 (15, 0) -> (15, 12) construction
  line L6 (15, 12) -> (0, 12) construction
  line L7 (0, 12) -> (0, 0) construction
  dimension "d5" = 5
  dimension "d8" = 0
  text T0 "12 V" font "Arial" height 5 align centre middle in box 15 x 12 at (0, 0) x (1, 0) y (0, 1) spacing 1 kerned
  constraint coincident L2.end
  constraint coincident L0.end
extrude "Extrude2" add sketch "Text" along normal blind 0.01 separate body text T0 makes body 2 at (5.4445, 0, 3.6967) makes body 3 at (10.6139, 0, 7.2892) makes body 4 at (2.3602, 0, 6.4775)
equation "d8 = 12 V"

design "Savöx SH 0255 MG Micro Servo Horn"
Autodesk Fusion 360 part; units mm, degrees
sketch "Sketch1" plane through (0, 0, 0) normal (0, 0, 1) x (1, 0, 0)
  circle A0 centre (0, 0) radius 12
  dimension "d1" = 24
  constraint coincident A0.centre origin
  measures "d1" diameter of A0
extrude "Extrude1" add sketch "Sketch1" along normal blind 2
sketch "Sketch2" plane through (0, 0, 0) normal (0, 0, -1) x (1, 0, 0)
  circle A0 centre (0, 0) radius 12
  circle A1 centre (0, 0) radius 2.5
  circle A2 centre (0, 0) radius 3.5
  dimension "d4" = 5
  dimension "d5" = 7
  constraint concentric A0 A1
  constraint concentric A1 A2
  measures "d4" diameter of A1
  measures "d5" diameter of A2
extrude "Extrude2" add sketch "Sketch2" along normal blind 2 contours A2

design "Sorted Smarties Cover Connector Clip"
Autodesk Fusion 360 part; units mm, degrees
sketch "Sorted Smarties Cover Connector Clip" plane through (0, 0, 0) normal (0, 0, 1) x (1, 0, 0)
  line L0 (0, 0) -> (24, 0)
  line L1 (24, 0) -> (24, 17)
  line L2 (24, 17) -> (0, 17)
  line L3 (0, 17) -> (0, 0)
  dimension "d6" = 24
  dimension "d7" = 17
  constraint horizontal L0
  constraint vertical L1
  constraint horizontal L2
  constraint vertical L3
  constraint coincident L0.start L3.end
  measures "d6" distance of L0.start L0.end
  measures "d7" distance of L0.end L1.end
extrude "Extrude1" add sketch "Sorted Smarties Cover Connector Clip" along normal blind 4
sketch "Connecting Section" plane through (0, 0, 4) normal (0, 0, 1) x (-1, 0, 0)
  line L0 (0, -17) -> (0, 0)
  line L1 (0, 0) -> (-24, 0)
  line L2 (-24, 0) -> (-24, -17)
  line L3 (-24, -17) -> (0, -17)
  line L4 (0, -17) -> (-24, -17)
  line L5 (-24, -17) -> (-24, -12)
  line L6 (-24, -12) -> (0, -12)
  line L7 (0, -12) -> (0, -17)
  dimension "d5" = 5
  constraint horizontal L4
  constraint vertical L5
  constraint horizontal L6
  constraint vertical L7
  constraint coincident L2 L5.end
  constraint coincident L0.start L3.end
  measures "d5" distance of L2.end L5.end
extrude "Extrude2" add sketch "Connecting Section" along normal blind 9 contours L0 L2 L3 L4 L5 L6 L7
sketch "Sorted Smarties Cover Section" plane through (0, 0, 4) normal (0, 0, 1) x (-1, 0, 0)
  line L0 (-24, -12) -> (0, -12)
  line L1 (0, -12) -> (0, 0)
  line L2 (0, 0) -> (-24, 0)
  line L3 (-24, 0) -> (-24, -12)
  line L4 (0, 0) -> (-24, 0)
  line L5 (-24, 0) -> (-24, -4)
  line L6 (-24, -4) -> (0, -4)
  line L7 (0, -4) -> (0, 0)
  dimension "d8" = 4
  constraint horizontal L4
  constraint vertical L5
  constraint horizontal L6
  constraint vertical L7
  constraint coincident L3 L5.end
  constraint coincident L1.end L2.start
  measures "d8" distance of L4 L6
extrude "Extrude3" add sketch "Sorted Smarties Cover Section" along normal blind 15 contours L1 L2 L3 L4 L5 L6 L7
move_body "Move1" bodies 1 to x (-1, 0, 0) y (0, -1, 0) z (0, 0, 1) at (24, 17, 0)

design "Sorted Smarties Cover"
Autodesk Fusion 360 part; units mm, degrees
sketch "Sketch1" plane through (0, 0, 0) normal (0, 1, 0) x (1, 0, 0)
  line L0 (0, 0) -> (270, 0)
  line L1 (270, 0) -> (270, -264)
  line L2 (270, -264) -> (0, -264)
  line L3 (0, -264) -> (0, 0)
  dimension "d1" = 270
  dimension "d2" = 264
  constraint horizontal L0
  constraint vertical L1
  constraint horizontal L2
  constraint vertical L3
  constraint coincident L0.start L3.end
  measures "d1" distance of L1.end L2.end
  measures "d2" distance of L0.end L1.end
extrude "Extrude1" add sketch "Sketch1" along normal blind 6
sketch "Sketch2" plane through (0, 0, 0) normal (0, -1, 0) x (1, 0, 0)
  line L0 (270, 264) -> (0, 264)
  line L1 (0, 264) -> (0, 0)
  line L2 (0, 0) -> (270, 0)
  line L3 (270, 0) -> (270, 264)
  line L4 (25.625, 231.1665) -> (43.625, 231.1665)
  line L5 (43.625, 231.1665) -> (43.625, 213.1665)
  line L6 (43.625, 213.1665) -> (25.625, 213.1665)
  line L7 (25.625, 213.1665) -> (25.625, 231.1665)
  line L8 (91.875, 231.1665) -> (109.875, 231.1665)
  line L9 (109.875, 231.1665) -> (109.875, 213.1665)
  line L10 (109.875, 213.1665) -> (91.875, 213.1665)
  line L11 (91.875, 213.1665) -> (91.875, 231.1665)
  line L12 (160.125, 231.1665) -> (178.125, 231.1665)
  line L13 (178.125, 231.1665) -> (178.125, 213.1665)
  line L14 (178.125, 213.1665) -> (160.125, 213.1665)
  line L15 (160.125, 213.1665) -> (160.125, 231.1665)
  line L16 (226.375, 231.1665) -> (244.375, 231.1665)
  line L17 (244.375, 231.1665) -> (244.375, 213.1665)
  line L18 (244.375, 213.1665) -> (226.375, 213.1665)
  line L19 (226.375, 213.1665) -> (226.375, 231.1665)
  line L20 (25.625, 111.6665) -> (43.625, 111.6665)
  line L21 (43.625, 111.6665) -> (43.625, 93.6665)
  line L22 (43.625, 93.6665) -> (25.625, 93.6665)
  line L23 (25.625, 93.6665) -> (25.625, 111.6665)
  line L24 (91.875, 111.6665) -> (109.875, 111.6665)
  line L25 (109.875, 111.6665) -> (109.875, 93.6665)
  line L26 (109.875, 93.6665) -> (91.875, 93.6665)
  line L27 (91.875, 93.6665) -> (91.875, 111.6665)
  line L28 (160.125, 111.6665) -> (178.125, 111.6665)
  line L29 (178.125, 111.6665) -> (178.125, 93.6665)
  line L30 (178.125, 93.6665) -> (160.125, 93.6665)
  line L31 (160.125, 93.6665) -> (160.125, 111.6665)
  line L32 (226.375, 111.6665) -> (244.375, 111.6665)
  line L33 (244.375, 111.6665) -> (244.375, 93.6665)
  line L34 (244.375, 93.6665) -> (226.375, 93.6665)
  line L35 (226.375, 93.6665) -> (226.375, 111.6665)
  dimension "d5" = 18
  dimension "d6" = 18
  dimension "d7" = 18
  dimension "d8" = 18
  dimension "d9" = 18
  dimension "d10" = 18
  dimension "d11" = 270
  dimension "d12" = 264
  dimension "d13" = 25.625
  dimension "d17" = 32.8335
  dimension "d18" = 152.3335
  dimension "d19" = 48.25
  dimension "d22" = 48.25
  dimension "d24" = 25.625
  constraint horizontal L4
  constraint vertical L5
  constraint horizontal L6
  constraint vertical L7
  constraint horizontal L8
  constraint vertical L9
  constraint horizontal L10
  constraint vertical L11
  constraint horizontal L12
  constraint vertical L13
  constraint horizontal L14
  constraint vertical L15
  constraint horizontal L16
  constraint vertical L17
  constraint horizontal L18
  constraint vertical L19
  constraint collinear L12 L16
  constraint collinear L8 L12
  constraint collinear L4 L8
  constraint collinear L14 L18
  constraint collinear L10 L14
  constraint collinear L6 L10
  constraint horizontal L20
  constraint vertical L21
  constraint horizontal L22
  constraint vertical L23
  constraint horizontal L24
  constraint vertical L25
  constraint horizontal L26
  constraint vertical L27
  constraint horizontal L28
  constraint vertical L29
  constraint horizontal L30
  constraint vertical L31
  constraint horizontal L32
  constraint vertical L33
  constraint horizontal L34
  constraint vertical L35
  constraint collinear L7 L23
  constraint collinear L5 L21
  constraint collinear L11 L27
  constraint collinear L9 L25
  constraint collinear L15 L31
  constraint collinear L13 L29
  constraint collinear L19 L35
  constraint collinear L17 L33
  constraint collinear L20 L24
  constraint collinear L24 L28
  constraint collinear L28 L32
  constraint collinear L22 L26
  constraint collinear L26 L30
  constraint collinear L30 L34
  measures "d5" distance of L5.end L6.end
  measures "d6" distance of L9.end L10.end
  measures "d7" distance of L13.end L14.end
  measures "d8" distance of L17.end L18.end
  measures "d9" distance of L4.start L6.end
  measures "d10" distance of L20.start L22.end
  measures "d11" distance of L0.start L0.end
  measures "d12" distance of L0.start L2.end
  measures "d13" distance of L1 L7
  measures "d17" distance of L0 L4
  measures "d18" distance of L0 L20
  measures "d19" distance of L5 L11
  measures "d22" distance of L13 L19
  measures "d24" distance of L3 L17
extrude "Extrude2" cut sketch "Sketch2" against normal blind 6 contours L4 L5 L6 L7 | L8 L9 L10 L11 | L12 L13 L14 L15 | L16 L17 L18 L19 | L20 L21 L22 L23 | L24 L25 L26 L27 | L28 L29 L30 L31 | L32 L33 L34 L35
equation "d13 = 3 mm + ( ( 63.25 / 2 ) * 1 mm ) - ( ( 18 / 2 ) * 1 mm )"
equation "d17 = 3 mm + ( ( 77.667 / 2 ) * 1 mm ) - ( ( 18 / 2 ) * 1 mm )"
equation "d18 = 122.5 mm + ( ( 77.667 / 2 ) * 1 mm ) - ( ( 18 / 2 ) * 1 mm )"
equation "d19 = 3 mm + 63.25 mm - 18 mm"
equation "d22 = 3 mm + 63.25 mm - 18 mm"
equation "d24 = 3 mm + ( ( 63.25 / 2 ) * 1 mm ) - ( ( 18 / 2 ) * 1 mm )"

design "Smartie Feed"
Autodesk Fusion 360 part; units mm, degrees
sketch "Smartie Feed" plane through (0, 0, 0) normal (0, 0, 1) x (1, 0, 0)
  line L0 (0, 0) -> (209, 0)
  line L1 (209, 0) -> (209, 21)
  line L2 (209, 21) -> (0, 21)
  line L3 (0, 21) -> (0, 0)
  dimension "d1" = 209
  dimension "d2" = 21
  constraint horizontal L0
  constraint vertical L1
  constraint horizontal L2
  constraint vertical L3
  constraint coincident L0.start L3.end
  measures "d1" distance of L0.start L0.end
  measures "d2" distance of L0.end L1.end
extrude "Extrude1" add sketch "Smartie Feed" along normal blind 187
sketch "Outlet" plane through (0, 0, 0) normal (0, -1, 0) x (1, 0, 0)
  line L0 (0, 0) -> (209, 0)
  line L1 (209, 0) -> (209, 187)
  line L2 (209, 187) -> (0, 187)
  line L3 (0, 187) -> (0, 0)
  line L4 (69, 146) -> (159, 146)
  line L5 (159, 146) -> (159, 116)
  line L6 (159, 116) -> (69, 116)
  line L7 (69, 116) -> (69, 146)
  dimension "d31" = 30
  dimension "d32" = 90
  dimension "d33" = 69
  dimension "d34" = 50
  dimension "d35" = 41
  constraint horizontal L4
  constraint vertical L5
  constraint horizontal L6
  constraint vertical L7
  measures "d31" distance of L4.end L5.end
  measures "d32" distance of L4.start L4.end
  measures "d33" distance of L3 L7
  measures "d34" distance of L1 L5
  measures "d35" distance of L2 L4
sketch "Inlet" plane through (0, 21, 0) normal (0, 1, 0) x (-1, 0, 0)
  line L0 (-209, 0) -> (0, 0)
  line L1 (0, 0) -> (0, 187)
  line L2 (0, 187) -> (-209, 187)
  line L3 (-209, 187) -> (-209, 0)
  line L4 (-69, 152) -> (-159, 152)
  line L5 (-159, 152) -> (-159, 122)
  line L6 (-159, 122) -> (-69, 122)
  line L7 (-69, 122) -> (-69, 152)
  dimension "d36" = 90
  dimension "d37" = 69
  dimension "d38" = 30
  dimension "d39" = 35
  dimension "d40" = 50
  constraint horizontal L4
  constraint vertical L5
  constraint horizontal L6
  constraint vertical L7
  measures "d36" distance of L4.start L4.end
  measures "d37" distance of L1 L7
  measures "d38" distance of L4.start L6.end
  measures "d39" distance of L2 L4
  measures "d40" distance of L3 L5
loft "Loft9" cut profiles "Inlet", "Outlet" section 1 contours L4 L5 L6 L7 section 2 contours L4 L5 L6 L7
sketch "Sketch6" plane through (0, 21, 0) normal (0, 1, 0) x (-1, 0, 0)
  line L0 (-69, 152) -> (-69, 122)
  line L1 (-69, 122) -> (-159, 122)
  line L2 (-159, 122) -> (-159, 152)
  line L3 (-159, 152) -> (-69, 152)
  line L4 (-209, 0) -> (0, 0)
  line L5 (0, 0) -> (0, 187)
  line L6 (0, 187) -> (-209, 187)
  line L7 (-209, 187) -> (-209, 0)
  circle A0 centre (-164, 172) radius 2.75
  circle A1 centre (-64, 172) radius 2.75
  circle A2 centre (-164, 102) radius 2.75
  circle A3 centre (-64, 102) radius 2.75
  dimension "d43" = 5.5
  dimension "d44" = 5.5
  dimension "d45" = 5.5
  dimension "d46" = 5.5
  dimension "d49" = 64
  dimension "d50" = 64
  dimension "d51" = 164
  dimension "d52" = 164
  dimension "d53" = 20
  dimension "d54" = 20
  dimension "d55" = 20
  dimension "d56" = 20
  measures "d43" diameter of A0
  measures "d44" diameter of A2
  measures "d45" diameter of A1
  measures "d46" diameter of A3
  measures "d49" distance of L5 A1.centre
  measures "d50" distance of L5 A3.centre
  measures "d51" distance of L5 A0.centre
  measures "d52" distance of L5 A2.centre
  measures "d53" distance of L3 A1.centre
  measures "d54" distance of L3 A0.centre
  measures "d55" distance of L1 A2.centre
  measures "d56" distance of L1 A3.centre
extrude "Extrude2" cut sketch "Sketch6" against normal blind 1.5 contours A0 | A1 | A2 | A3
equation "d1 = 219 mm - 10 mm"
equation "d3 = 166 mm + 21 mm"
equation "outletHeight = 15 mm"
equation "outletWidth = 20 mm"
equation "sortedContainersMidpointWidth = sortedContainersWidth + polycarbonateThickness"
equation "sortedContainersWidth = 60 mm"
equation "sortedContainersHeight = 113 mm"
equation "polycarbonateThickness = 6 mm"
equation "sortedContainersMidpointHeight = sortedContainersHeight + polycarbonateThickness"
equation "d33 = 90 mm - 21 mm"
equation "d35 = 30 mm - 21 mm + 5 mm + 6 mm + 21 mm"
equation "d37 = 90 mm - 21 mm"
equation "d39 = 30 mm - 21 mm + 5 mm + 21 mm"
equation "magnetDiameter = 5 mm"
equation "magnetHeight = 1.5 mm"
equation "d43 = magnetDiameter + 0.5 mm"
equation "d44 = magnetDiameter + 0.5 mm"
equation "d45 = magnetDiameter + 0.5 mm"
equation "d46 = magnetDiameter + 0.5 mm"
equation "d49 = 75 mm - 21 mm + 10 mm"
equation "d50 = 75 mm - 21 mm + 10 mm"
equation "d51 = 195 mm - 10 mm - 21 mm"
equation "d52 = 195 mm - 10 mm - 21 mm"

design "Back Panel Support Right"
Autodesk Fusion 360 part; units mm, degrees
sketch "Back Panel Support Left " plane through (0, 0, 0) normal (1, 0, 0) x (0, 1, 0)
  line L0 (0, 0) -> (21, 0)
  line L1 (21, 0) -> (21, 270)
  line L2 (21, 270) -> (0, 270)
  line L3 (0, 270) -> (0, 0)
  dimension "d1" = 270
  dimension "d2" = 21
  constraint horizontal L0
  constraint vertical L1
  constraint horizontal L2
  constraint vertical L3
  constraint coincident L0.start L3.end
  measures "d1" distance of L0.end L1.end
  measures "d2" distance of L0.start L0.end